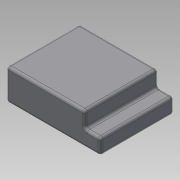
# Autodesk Inventor part: battery
Saved by Autodesk Inventor 2015 SP1 (Build 190203100, 203)
## iProperties
Created: 2015-01-05
Part Number: battery
Material: Generic
Document SubType Name: Modeling
Designer: Mathieu
Density: 1 g/cm^3
Appearance: Default
Mass: 1.37806 g
Surface Area: 8.31273 cm^2
Volume: 1.37806 cm^3
Author: Mathieu
Autodesk Inventor part; units mm, degrees
ref_plane "YZ Plane" through (0, 0, 0) normal (1, 0, 0) x (0, 1, 0)
ref_plane "XZ Plane" through (0, 0, 0) normal (0, 1, 0) x (-1, 0, 0)
ref_plane "XY Plane" through (0, 0, 0) normal (0, 0, 1) x (1, 0, 0)
sketch "Sketch1" plane through (0, 0, 0) normal (0, 0, 1) x (1, 0, 0)
  line L0 (0, 0) -> (18, 0)
  line L1 (18, 0) -> (18, 14)
  line L2 (18, 14) -> (0, 14)
  line L3 (0, 14) -> (0, 0)
  dimension "d0" = 18
  dimension "d1" = 14
  constraints: 8 end point, 2 parallel, 1 horizontal, 1 perpendicular
  measures "d0" distance of L1.end L2.end
  measures "d1" distance of L0.end L1.end
extrude "Extrusion1" add sketch "Sketch1" along normal blind 6
sketch "Sketch2" plane through (0, 0, 0) normal (0, -1, 0) x (1, 0, 0)
  line L0 (18, 6) -> (15, 6)
  line L1 (15, 6) -> (15, 3)
  line L2 (15, 3) -> (18, 3)
  line L3 (18, 3) -> (18, 6)
  point P0 (0, 0)
  dimension "d5" = 3
  dimension "d6" = 3
  constraints: 8 end point, 2 parallel, 1 horizontal, 1 perpendicular
  measures "d5" distance of L1.end L2.end
  measures "d6" distance of L0.end L1.end
extrude "Extrusion2" cut sketch "Sketch2" against normal up to next
fillet "Fillet1" radius 0.5 18 edges at (0, 7, 0) (0, 0, 3) (0, 7, 6) (0, 14, 3) (9, 14, 0) (7.5, 14, 6) (18, 14, 1.5) (18, 7, 0) (18, 0, 1.5) (9, 0, 0) (7.5, 0, 6) (15, 7, 3) (15, 7, 6) (15, 0, 4.5) (16.5, 0, 3) (16.5, 14, 3) (18, 7, 3) (15, 14, 4.5)
body "Solid1"
